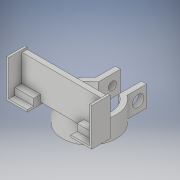
# Autodesk Inventor part: Ultrasonic Mount
Saved by Autodesk Inventor 2018 (Build 220112000, 112)
## iProperties
Created: 2018-01-09
Part Number: Ultrasonic Mount
Material: Generic
Document SubType Name: Modeling
Designer: prakh
Density: 1 g/cm^3
Appearance: Default
Author: prakh
Autodesk Inventor part; units mm, degrees
ref_plane "YZ Plane" through (0, 0, 0) normal (1, 0, 0) x (0, 1, 0)
ref_plane "XZ Plane" through (0, 0, 0) normal (0, 1, 0) x (-1, 0, 0)
ref_plane "XY Plane" through (0, 0, 0) normal (0, 0, 1) x (1, 0, 0)
sketch "Sketch1" plane through (0, 0, 0) normal (0, 0, 1) x (1, 0, 0)
  arc A0 (11.726, 6.35) -> (11.726, -6.35) centre (0, 0) ccw
  line L0 (25.4, -9.525) -> (13.4853, -9.525)
  line L1 (6.1638, -4.445) -> (6.1638, -1.27)
  line L2 (11.726, -6.35) -> (25.4, -6.35)
  line L3 (25.4, -6.35) -> (25.4, -9.525)
  line L4 (25.4, 6.35) -> (11.726, 6.35)
  line L5 (8.3094, 1.6345) -> (8.3094, 4.8095)
  line L6 (25.4, 9.525) -> (25.4, 6.35)
  line L7 (13.4853, 9.525) -> (25.4, 9.525)
  arc A1 (13.4853, 9.525) -> (13.4853, -9.525) centre (0, 0) ccw
  dimension "d0" = 26.67
  dimension "d2" = 3.175
  dimension "d3" = 9.525
  dimension "d4" = 25.4
  dimension "d5" = 3.175
  constraints: 16 end point, 4 parallel, 4 point on circle, 2 centre point, 2 coincident, 2 equal length, 2 horizontal, 2 perpendicular, 1 collinear
  measures "d0" diameter of A0
  measures "d2" distance of L2.end L0.start
  measures "d3" distance from line of point (0, 0) L0
  measures "d4" distance from line of point (0, 0) L3
  measures "d5" radial gap between concentric circles of A0 A1
extrude "Extrusion1" add sketch "Sketch1" along normal blind 12.7
sketch "Sketch2" plane through (13.4853, 9.525, 0) normal (0, 1, 0) x (1, 0, 0)
  circle A0 centre (6.8347, -6.35) radius 2.4638
  line L0 (11.9147, -12.7) -> (0, -12.7) projected
  line L1 (11.9147, 0) -> (11.9147, -12.7) projected
  point P0 (-13.4853, 0)
  dimension "d8" = 6.35
  dimension "d9" = 5.08
  dimension "d10" = 4.9276
  constraints: 1 centre point
  measures "d8" distance from line of A0.centre L0
  measures "d9" distance from line of A0.centre L1
  measures "d10" diameter of A0
extrude "Extrusion2" cut sketch "Sketch2" against normal blind 25.4
sketch "Sketch3" plane through (13.4853, 9.525, 0) normal (0, 1, 0) x (1, 0, 0)
  circle A0 centre (6.8347, -6.35) radius 2.4638 projected
  circle A1 centre (6.8347, -6.35) radius 3.4798
  point P0 (-13.4853, 0)
  dimension "d13" = 1.016
  constraints: 1 centre point, 1 coincident
  measures "d13" radial gap between concentric circles of A0 A1
extrude "Extrusion3" cut sketch "Sketch3" against normal up to surface (3.175 mm away)
sketch "Sketch4" plane through (0, 0, 0) normal (0, 0, -1) x (-1, 0, 0)
  line L0 (16.51, -24.765) -> (13.335, -24.765)
  line L1 (13.335, -24.765) -> (13.335, 24.765)
  line L2 (13.335, 24.765) -> (16.51, 24.765)
  line L3 (16.51, 24.765) -> (16.51, -24.765)
  arc A0 (-11.726, -6.35) -> (-11.726, 6.35) centre (0, 0) ccw projected
  arc A1 (-13.4853, -9.525) -> (-13.4853, 9.525) centre (0, 0) ccw projected
  dimension "d20" = 49.53
  dimension "d21" = 24.765
  constraints: 8 end point, 2 parallel, 2 tangent, 1 horizontal, 1 perpendicular
  measures "d20" distance between parallel lines of L0 L2
  measures "d21" distance from line of point (0, 0) L0
extrude "Extrusion4" add sketch "Sketch4" along normal blind 20.6375
sketch "Sketch5" plane through (-13.335, -24.765, 0) normal (1, 0, 0) x (0, 0, -1)
  line L0 (21.9075, -1.27) -> (-1.27, -1.27)
  line L1 (-1.27, 50.8) -> (21.9075, 50.8)
  line L2 (0, 49.53) -> (20.6375, 49.53) projected
  line L3 (0, 34.4994) -> (0, 49.53) projected
  line L4 (0, 0) -> (20.6375, 0) projected
  line L5 (20.6375, 0) -> (0, 0)
  line L6 (0, 49.53) -> (20.6375, 49.53)
  line L7 (20.6375, 49.53) -> (21.9075, 49.53)
  line L8 (20.6375, 0) -> (21.9075, 0)
  line L9 (0, 38.1) -> (-1.27, 38.1)
  line L10 (0, 11.43) -> (-1.27, 11.43)
  line L11 (21.9075, 50.8) -> (21.9075, 49.53)
  line L12 (21.9075, 0) -> (21.9075, -1.27)
  line L13 (-1.27, -1.27) -> (-1.27, 11.43)
  line L14 (-1.27, 38.1) -> (-1.27, 50.8)
  line L15 (0, 0) -> (0, 11.43)
  line L16 (0, 38.1) -> (0, 49.53)
  point P0 (0, 24.765)
  dimension "d22" = 1.27
  dimension "d24" = 1.27
  dimension "d28" = 23.1775
  dimension "d29" = 12.7
  dimension "d30" = 1.27
  dimension "d31" = 1.27
  constraints: 28 end point, 6 horizontal, 6 parallel, 4 perpendicular, 2 equal length, 1 collinear
  measures "d22" distance between parallel lines of L1 L2
  measures "d24" distance between parallel lines of L0 L4
  measures "d28" distance of L1.start L1.end
  measures "d29" distance of L9.end L1.start
  measures "d30" distance between parallel lines of L3 L14
  measures "d31" distance between parallel lines of L15 L13
extrude "Extrusion5" add sketch "Sketch5" against normal blind 11.303
sketch "Sketch7" plane through (-16.51, -13.335, 0) normal (-1, 0, 0) x (0, 0, 1)
  line L0 (0, 38.1) -> (0, 26.67) projected
  line L1 (0, 38.1) -> (-20.6375, 38.1) projected
  line L2 (-20.6375, -11.43) -> (-20.6375, 38.1) projected
  line L3 (0, -11.43) -> (-20.6375, -11.43) projected
  line L4 (0, 0) -> (0, -11.43) projected
  line L5 (0, 13.335) -> (0, 0) projected
  line L6 (0, 26.67) -> (0, 13.335) projected
  line L7 (0, -11.43) -> (-4.114, -11.43)
  line L8 (-4.114, -11.43) -> (-4.114, 0)
  line L9 (-4.114, 0) -> (0, 0)
  line L10 (0, 0) -> (0, -11.43)
  line L11 (0, 38.1) -> (-4.114, 38.1)
  line L12 (-4.114, 38.1) -> (-4.114, 26.67)
  line L13 (-4.114, 26.67) -> (0, 26.67)
  line L14 (0, 26.67) -> (0, 38.1)
  constraints: 16 end point, 4 parallel, 2 horizontal, 2 perpendicular, 1 point on line
extrude "Extrusion7" add sketch "Sketch7" along normal blind 4.318 contours L0 L13 L12 L1 | L4 L3 L8 L9
equation "\"d21\" = 0.5 * d20"
equation "\"d24\" = d22"
equation "\"d30\" = d22"
equation "\"d31\" = d22"
equation "\"d23\" = d22"
equation "\"d25\" = d22"
body "Solid1"
